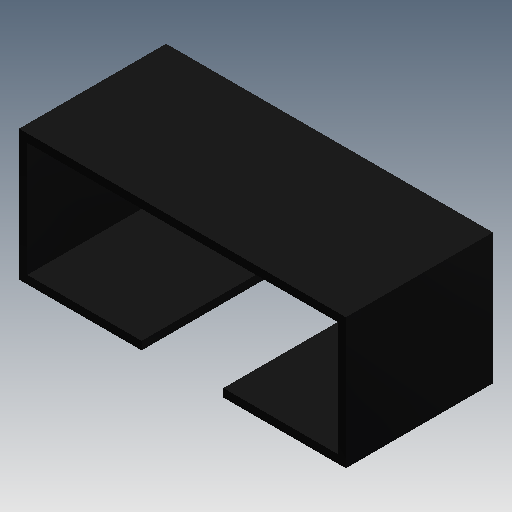
# Autodesk Inventor part: config - c9g5 connector
Saved by Autodesk Inventor 2020 (Build 240152000, 152)
## iProperties
Created: 2005-12-05
Part Number: config - c9g5 connector
Document SubType Name: Modeling
Designer: Simon.Ng@autodesk.com
Stock Number: config - c9g5 connector
Density: 1 g/cm^3
Material: Generic
Mass: 0.28825 g
Surface Area: 11.895 cm^2
Volume: 0.28825 cm^3
Appearance: Glossy - Black
Company: Autodesk Asia Pte. Ltd.
Title: PC Demo
Author: Simon.Ng@autodesk.com
Autodesk Inventor part; units mm, degrees
ref_plane "YZ Plane" through (0, 0, 0) normal (1, 0, 0) x (0, 1, 0)
ref_plane "XZ Plane" through (0, 0, 0) normal (0, 1, 0) x (-1, 0, 0)
ref_plane "XY Plane" through (0, 0, 0) normal (0, 0, 1) x (1, 0, 0)
sketch "Sketch1" plane through (0, 0, 0) normal (0, 0, 1) x (1, 0, 0)
  line L0 (0, 6.4) -> (0, -4.8) projected
  line L1 (-12, 0) -> (16, 0) projected
  line L2 (-10, 4) -> (10, 4)
  line L3 (10, 4) -> (10, -4)
  line L4 (10, -4) -> (-10, -4)
  line L5 (-10, -4) -> (-10, 4)
  dimension "d0" = 20
  dimension "d1" = 8
  constraints: 8 end point, 2 parallel, 1 horizontal, 1 perpendicular, 2 other
  measures "d0" distance of L3.end L4.end
  measures "d1" distance of L4.end L2.start
extrude "Extrusion1" add sketch "Sketch1" along normal blind 9
shell "Shell1" thickness 0.5 removed faces 1 at (3.3333, -1.3333, 9)
sketch "Sketch2" plane through (-10, -4, 0) normal (0, -1, 0) x (1, 0, 0)
  line L0 (20, 9) -> (0, 9) construction
  line L1 (19.5, 0.5) -> (0.5, 0.5) construction
  line L2 (10, 11.7) -> (10, -0.9) construction
  line L3 (7.5, 9) -> (12.5, 9)
  line L4 (12.5, 9) -> (12.5, 0.5)
  line L5 (12.5, 0.5) -> (7.5, 0.5)
  line L6 (7.5, 0.5) -> (7.5, 9)
  dimension "d5" = 5
  constraints: 8 end point, 2 parallel, 2 point on line, 1 horizontal, 1 perpendicular, 1 other
  measures "d5" distance between parallel lines of L4 L6
extrude "Extrusion2" cut sketch "Sketch2" against normal up to next
body "Solid1"
